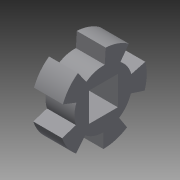
# Autodesk Inventor part: SmallGear
Saved by Autodesk Inventor 2015 (Build 190159000, 159)
## iProperties
Created: 2015-06-16
Part Number: SmallGear
Material: Generic
Document SubType Name: Modeling
Designer: david_000
Density: 1 g/cm^3
Appearance: Default
Author: david_000
Autodesk Inventor part; units mm, degrees
ref_plane "YZ Plane" through (0, 0, 0) normal (1, 0, 0) x (0, 1, 0)
ref_plane "XZ Plane" through (0, 0, 0) normal (0, 1, 0) x (-1, 0, 0)
ref_plane "XY Plane" through (0, 0, 0) normal (0, 0, 1) x (1, 0, 0)
sketch "Sketch2" plane through (0, 0, 0) normal (1, 0, 0) x (0, 1, 0)
  line L0 (0, 0) -> (1.27, 0)
  line L1 (1.27, 0) -> (1.27, -1.27)
  line L2 (1.27, -1.27) -> (0, -1.27)
  line L3 (0, -1.27) -> (0, 0)
  circle A0 centre (0.635, -0.635) radius 1.27
  line L4 (-0.4301, -1.3267) -> (-0.9627, -1.6725)
  line L5 (-0.635, -0.635) -> (-1.27, -0.635)
  arc A1 (0.0463, -2.4468) -> (1.1281, -2.4751) centre (0.635, -0.635) ccw
  arc A2 (2.1762, -1.7547) -> (2.5374, -0.7347) centre (0.635, -0.635) ccw
  arc A3 (2.1762, 0.4847) -> (1.3177, 1.1435) centre (0.635, -0.635) ccw
  arc A4 (0.0463, 1.1768) -> (-0.8455, 0.5639) centre (0.635, -0.635) ccw
  arc A5 (-1.27, -0.635) -> (-0.9627, -1.6725) centre (0.635, -0.635) ccw
  line L6 (0.6317, -0.6225) -> (0.8051, -1.27)
  line L7 (0.9637, -1.8617) -> (1.1281, -2.4751)
  line L8 (0.0463, -2.4468) -> (0.2403, -1.8421)
  line L9 (0.4239, -1.27) -> (0.6317, -0.6225)
  line L10 (1.3177, 1.1435) -> (1.0878, 0.5516)
  line L11 (0.8735, 0) -> (0.6317, -0.6225)
  line L12 (2.1762, 0.4847) -> (1.6601, 0.1147)
  line L13 (1.27, -0.1649) -> (0.6317, -0.6225)
  line L14 (2.5374, -0.7347) -> (1.9035, -0.6974)
  line L15 (1.27, -0.6601) -> (0.6317, -0.6225)
  line L16 (2.1762, -1.7547) -> (1.664, -1.3793)
  line L17 (1.27, -1.0905) -> (0.6317, -0.6225)
  line L18 (0.0463, 1.1768) -> (0.2428, 0.5729)
  line L19 (0.4291, 0) -> (0.6317, -0.6225)
  line L20 (-0.8455, 0.5639) -> (-0.3504, 0.1662)
  line L21 (0, -0.1152) -> (0.6317, -0.6225)
  dimension "d15" = 2.54
  dimension "d13" = 1.27
  dimension "d14" = 1.27
  constraints: 44 end point, 10 point on circle, 8 point on line, 5 centre point, 2 horizontal, 2 parallel, 1 coincident, 1 perpendicular, 12 other
  measures "d13" distance of L1.end L2.end
  measures "d14" distance of L0.end L1.end
extrude "Extrusion2" add sketch "Sketch2" along normal blind 1.27
body "Solid2"
